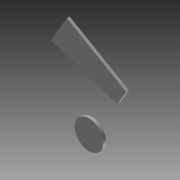
# Autodesk Inventor part: mean machine brow
Saved by Autodesk Inventor 2012 (Build 160160000, 160)
## iProperties
Created: 2013-12-19
Part Number: mean machine brow
Material: Default
Document SubType Name: Modeling
Designer: Bryce
Density: 1 g/cm^3
Author: Bryce
Autodesk Inventor part; units mm, degrees
ref_plane "YZ Plane" through (0, 0, 0) normal (1, 0, 0) x (0, 1, 0)
ref_plane "XZ Plane" through (0, 0, 0) normal (0, 1, 0) x (-1, 0, 0)
ref_plane "XY Plane" through (0, 0, 0) normal (0, 0, 1) x (1, 0, 0)
sketch "Sketch1" plane through (0, 0, 0) normal (0, 0, 1) x (1, 0, 0)
  circle A0 centre (0, 0) radius 15.875
  line L0 (18.3309, 31.75) -> (36.6617, 0) construction
  line L1 (36.6617, 0) -> (18.3309, -31.75) construction
  line L2 (18.3309, -31.75) -> (-18.3309, -31.75) construction
  line L3 (-18.3309, -31.75) -> (-36.6617, 0) construction
  line L4 (-36.6617, 0) -> (-18.3309, 31.75) construction
  line L5 (-18.3309, 31.75) -> (18.3309, 31.75) construction
  line L6 (-42.1786, 69.85) -> (31.75, 45.4982)
  line L7 (31.75, 45.4982) -> (41.275, 61.9959)
  line L8 (41.275, 61.9959) -> (-24.7161, 100.0959)
  line L9 (-24.7161, 100.0959) -> (-42.1786, 69.85)
  line L10 (0, 0) -> (69.4257, 0) construction
  dimension "d5" = 31.75
  dimension "d6" = 63.5
  dimension "d7" = 76.2
  dimension "d8" = 19.05
  dimension "d9" = 34.925
  dimension "d10" = 69.85
  dimension "d11" = 31.75
  constraints: 22 end point, 3 coincident, 2 horizontal, 2 perpendicular, 1 centre point, 1 parallel, 13 other
  measures "d5" diameter of A0
  measures "d6" distance between parallel lines of L2 L5
  measures "d7" distance of L7.end L8.end
  measures "d8" distance of L6.end L7.end
  measures "d9" distance of L8.end L6.start
  measures "d10" vertical distance of L6.start point (0, 0)
  measures "d11" horizontal distance of point (0, 0) L6.end
extrude "Extrusion1" add sketch "Sketch1" along normal blind 3.175
body "Solid1"
